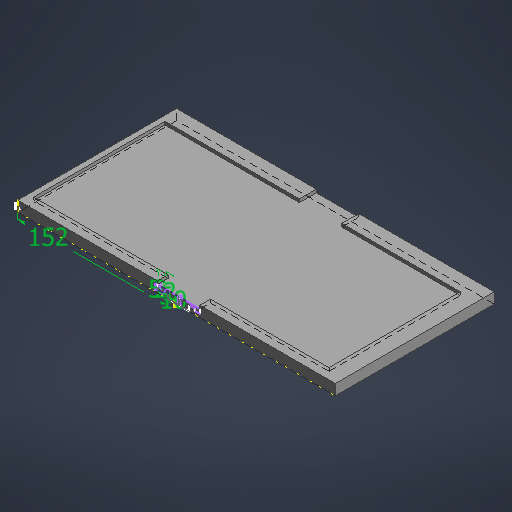
# Autodesk Inventor part: tray_multipart
Saved by Autodesk Inventor 2026 (Build 300175050, 175E)
## iProperties
Part Number: tray_multipart
Material: Generic
Document SubType Name: Modeling
Designer: romanov
Appearance: Default
Author: romanov
Autodesk Inventor part; units mm, degrees
ref_plane "YZ Plane" through (0, 0, 0) normal (1, 0, 0) x (0, 1, 0)
ref_plane "XZ Plane" through (0, 0, 0) normal (0, 1, 0) x (-1, 0, 0)
ref_plane "XY Plane" through (0, 0, 0) normal (0, 0, 1) x (1, 0, 0)
sketch "Sketch1" plane through (0, 0, 0) normal (0, 1, 0) x (-1, 0, 0)
  line L0 (150, 75) -> (-150, 75)
  line L1 (-150, 75) -> (-150, -75)
  line L2 (-150, -75) -> (150, -75)
  line L3 (150, -75) -> (150, 75)
  line L4 (150, 75) -> (-150, -75) construction
  line L5 (-150, 75) -> (150, -75) construction
  point P0 (0, 0)
  dimension "d0" = 300
  dimension "d1" = 150
  constraints: 12 end point, 2 midpoint, 2 parallel, 1 horizontal, 1 perpendicular
  measures "d0" distance between parallel lines of L1 L3
  measures "d1" distance between parallel lines of L0 L2
extrude "Extrusion1" add sketch "Sketch1" along normal blind 10
sketch "Sketch3" plane through (0, 10, 0) normal (0, 1, 0) x (1, 0, 0)
  line L0 (-145, -65) -> (134, -65)
  line L1 (134, -65) -> (134, 59)
  line L2 (134, 59) -> (-145, 59)
  line L3 (-145, 59) -> (-145, -65)
  line L4 (-150, 75) -> (-150, -75) projected
  line L5 (-150, -75) -> (150, -75) projected
  point P0 (0, 0)
  dimension "d4" = 279
  dimension "d5" = 124
  dimension "d6" = 5
  dimension "d7" = 10
  constraints: 8 end point, 2 parallel, 1 horizontal, 1 perpendicular
  measures "d4" distance of L1.end L2.end
  measures "d5" distance of L0.end L1.end
  measures "d6" distance between parallel lines of L4 L3
  measures "d7" distance between parallel lines of L5 L0
extrude "Extrusion2" cut sketch "Sketch3" against normal blind 3
sketch "Sketch5" plane through (-150, 0, 75) normal (0, 0, 1) x (1, 0, 0)
  line L0 (300, 0) -> (0, 0) construction
  line L1 (152, 0) -> (152, 9.9509) construction
  line L2 (0, 0) -> (0, 10) projected
  line L3 (152, 0) -> (152, 7)
  line L4 (132, 7) -> (132, 3)
  line L5 (132, 3) -> (137, 3)
  line L6 (137, 3) -> (137, 5)
  line L7 (137, 5) -> (142, 5)
  line L8 (142, 5) -> (142, 0)
  line L9 (142, 0) -> (152, 0)
  line L10 (132, 7) -> (152, 7)
  line L11 (172, 7) -> (172, 3)
  line L12 (172, 3) -> (167, 3)
  line L13 (167, 3) -> (167, 5)
  line L14 (167, 5) -> (162, 5)
  line L15 (162, 5) -> (162, 0)
  line L16 (162, 0) -> (152, 0)
  line L17 (172, 7) -> (152, 7)
  point P0 (150, 0)
  point P1 (0, 5)
  point P2 (152, 4.9755)
  point P3 (152, 3.5)
  point P4 (137, 4)
  point P5 (132, 5)
  dimension "d15" = 152
  dimension "d16" = 10
  dimension "d17" = 5
  dimension "d18" = 5
  dimension "d19" = 2
  dimension "d20" = 2
  constraints: 32 end point, 6 symmetric about line, 5 midpoint, 4 perpendicular, 3 point on line, 1 collinear, 1 horizontal, 1 vertical
  measures "d15" distance of point (0, 5) point (152, 4.975)
  measures "d16" distance from line of point (152, 3.5) L8
  measures "d17" distance from line of L8 point (137, 4)
  measures "d18" distance from line of point (132, 5) L6
  measures "d19" distance between parallel lines of L10 L7
  measures "d20" distance between parallel lines of L7 L5
sketch "Sketch6" plane through (-150, 0, 75) normal (0, 0, 1) x (1, 0, 0)
  line L0 (5, 7) -> (284, 7) projected
  line L1 (300, 10) -> (0, 10) projected
  line L2 (132, 7) -> (171.9929, 7)
  line L3 (171.9929, 7) -> (171.9929, 10)
  line L4 (171.9929, 10) -> (132, 10)
  line L5 (132, 10) -> (132, 7)
  line L6 (132, 7) -> (132, 3) projected
  point P0 (150, 0)
  constraints: 8 end point, 3 point on line, 2 parallel, 1 collinear, 1 horizontal, 1 perpendicular
extrude "Extrusion3" cut sketch "Sketch6" against normal through all
equation "\"d4\" = pebble_width"
equation "\"d5\" = pebble_height"
equation "\"pebble_height\" = 124"
equation "\"pebble_width\" = 279"
equation "\"pebble_depth\" = 16"
body "Solid1"
